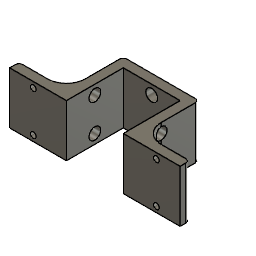
krep_karetka (Autodesk Fusion 360 design; units mm, degrees)
Autodesk Fusion 360 part; units mm, degrees
sketch "Sketch1" plane through (0, 0, 0) normal (0, 1, 0) x (1, 0, 0)
  line L0 (15, -15) -> (-15, -15)
  line L1 (-15, -15) -> (-15, 15)
  line L2 (-15, 15) -> (15, 15)
  line L3 (15, 15) -> (15, -15)
  line L4 (15, -15) -> (-15, 15) construction
  line L5 (-15, -15) -> (15, 15) construction
  line L6 (-15, -15) -> (-45, -15)
  line L7 (-45, -15) -> (-45, -10)
  line L8 (-45, -10) -> (-15, -10)
  line L9 (15, -15) -> (45, -15)
  line L10 (45, -15) -> (45, -10)
  line L11 (45, -10) -> (15, -10)
  line L12 (-15, 15) -> (-20, 15)
  line L13 (-20, 15) -> (-20, -10)
  line L14 (15, 15) -> (20, 15)
  line L15 (20, 15) -> (20, -10)
  line L16 (20, 15) -> (20, 20)
  line L17 (20, 20) -> (-20, 20)
  line L18 (-20, 20) -> (-20, 15)
  line L19 (-20, 20) -> (-45, -10)
  line L20 (20, 20) -> (45, -10)
  constraint horizontal L0
  constraint perpendicular L0 L1
  constraint parallel L0 L2
  constraint parallel L1 L3
  constraint coincident L4 origin
  constraint coincident L5 origin
  constraint perpendicular L1 L6
  constraint perpendicular L6 L7
  constraint coincident L1 L8.end
  constraint perpendicular L1 L8
  constraint perpendicular L3 L9
  constraint perpendicular L9 L10
  constraint coincident L3 L11.end
  constraint perpendicular L3 L11
  constraint perpendicular L1 L12
  constraint coincident L8 L13.end
  constraint perpendicular L8 L13
  constraint perpendicular L1 L14
  constraint coincident L11 L15.end
  constraint perpendicular L11 L15
  constraint perpendicular L14 L16
  constraint perpendicular L15 L17
  constraint perpendicular L12 L18
extrude "Extrude1" add sketch "Sketch1" along normal blind 27.5 contours L3 L9 L10 L11 | L1 L6 L7 L8 | L3 L11 L14 L15 | L1 L8 L12 L13 | L2 L12 L14 L16 L17 L18
sketch "Sketch2" plane through (0, 0, 15) normal (0, 0, 1) x (1, 0, 0)
  line L0 (-45, 0) -> (-15, 0)
  line L1 (-15, 0) -> (-15, 27.5)
  line L2 (-15, 27.5) -> (-45, 27.5)
  line L3 (-45, 27.5) -> (-45, 0)
  line L4 (0, 0) -> (0, 1.5209)
  circle A0 centre (-32.5, 24.5) radius 1.5
  circle A1 centre (-32.5, 3) radius 1.5
  circle A2 centre (32.5, 24.5) radius 1.5
  circle A3 centre (32.5, 3) radius 1.5
  dimension "d3" = 3
  dimension "d4" = 3
  dimension "d5" = 3
  dimension "d6" = 12.5
  dimension "d7" = 3
  dimension "d8" = 12.5
  constraint coincident L4.start origin
  constraint vertical L4
  constraint symmetric L4 A0 A2
  constraint symmetric L4 A1 A3
  measures "d3" diameter of A0
  measures "d4" diameter of A1
  measures "d5" distance of L2 A0.centre
  measures "d6" distance of L3 A0.centre
  measures "d7" distance of L0 A1.centre
  measures "d8" distance of L3 A1.centre
extrude "Extrude2" cut sketch "Sketch2" against normal blind 12 contours A0 | A1 | A2 | A3
sketch "Sketch3" plane through (20, 0, 0) normal (1, 0, 0) x (0, 0, -1)
  line L0 (-10, 0) -> (20, 0)
  line L1 (20, 0) -> (20, 27.5)
  line L2 (20, 27.5) -> (-10, 27.5)
  line L3 (-10, 27.5) -> (-10, 0)
  circle A0 centre (0, 22.5) radius 3.1
  circle A1 centre (0, 5) radius 3.1
  dimension "d11" = 6.2
  dimension "d24" = 5
  dimension "d25" = 5
  measures "d11" diameter of A0
  measures "d24" distance of L0 A1.centre
  measures "d25" distance of L2 A0.centre
extrude "Extrude3" cut sketch "Sketch3" against normal blind 68 contours A0 | A1
sketch "Sketch4" plane through (0, 0, -20) normal (0, 0, -1) x (-1, 0, 0)
  line L0 (-20, 0) -> (20, 0)
  line L1 (20, 0) -> (20, 27.5)
  line L2 (20, 27.5) -> (-20, 27.5)
  line L3 (-20, 27.5) -> (-20, 0)
  circle A0 centre (0, 22.5) radius 3.1
  circle A1 centre (0, 5) radius 3.1
  dimension "d14" = 6.2
  dimension "d15" = 6.2
  dimension "d26" = 5
  dimension "d27" = 5
  measures "d14" diameter of A0
  measures "d15" diameter of A1
  measures "d26" distance of L0 A1.centre
  measures "d27" distance of L2 A0.centre
extrude "Extrude4" cut sketch "Sketch4" against normal blind 12 contours A0 | A1
fillet "Fillet1" radius 10 2 edges at (20, 13.75, 10) (-20, 13.75, 10)
fillet "Fillet2" radius 2 2 edges at (20, 13.75, -20) (-20, 13.75, -20)
fillet "Fillet3" radius 2 2 edges at (45, 13.75, 10) (-45, 13.75, 10)
